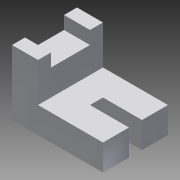
# Autodesk Inventor part: Aluminum
Saved by Autodesk Inventor 2015 (Build 190159000, 159)
## iProperties
Created: 2018-01-09
Part Number: Aluminum
Material: Aluminum 6061
Document SubType Name: Modeling
Designer: Administrator
Density: 2.7 g/cm^3
Appearance: Aluminum - Flat
Author: Administrator
Autodesk Inventor part; units mm, degrees
ref_plane "YZ Plane" through (0, 0, 0) normal (1, 0, 0) x (0, 1, 0)
ref_plane "XZ Plane" through (0, 0, 0) normal (0, 1, 0) x (-1, 0, 0)
ref_plane "XY Plane" through (0, 0, 0) normal (0, 0, 1) x (1, 0, 0)
sketch "Sketch1" plane through (0, 0, 0) normal (0, 0, 1) x (1, 0, 0)
  line L0 (0, 0) -> (0, 31.75)
  line L1 (0, 31.75) -> (12.7, 31.75)
  line L2 (12.7, 31.75) -> (12.7, 12.7)
  line L3 (12.7, 12.7) -> (44.45, 12.7)
  line L4 (44.45, 12.7) -> (44.45, 0)
  line L5 (44.45, 0) -> (0, 0)
  dimension "d0" = 31.75
  dimension "d1" = 44.45
  dimension "d2" = 19.05
  dimension "d3" = 12.7
  dimension "d4" = 12.7
  constraints: 12 end point, 4 perpendicular
  measures "d0" distance of L0.start L0.end
  measures "d1" distance of L4.end L0.start
  measures "d2" distance of L1.end L2.end
  measures "d3" distance of L0.end L1.end
  measures "d4" distance of L3.end L4.end
extrude "Extrusion1" add sketch "Sketch1" along normal blind 31.75
sketch "Sketch2" plane through (12.7, 12.7, 0) normal (1, 0, 0) x (0, 0, -1)
  line L0 (0, 19.05) -> (-31.75, 19.05) projected
  line L1 (-25.4, 19.05) -> (-25.4, 12.7)
  line L2 (-25.4, 12.7) -> (-6.35, 12.7)
  line L3 (-6.35, 12.7) -> (-6.35, 19.05)
  line L4 (-25.4, 19.05) -> (-6.35, 19.05)
  line L5 (-31.75, 0) -> (-31.75, 19.05) projected
  point P0 (0, -12.7)
  dimension "d7" = 6.35
  dimension "d8" = 19.05
  dimension "d9" = 6.35
  constraints: 8 end point, 4 perpendicular, 2 point on line
  measures "d7" distance of L2.end L3.end
  measures "d8" distance of L1.end L2.end
  measures "d9" distance between parallel lines of L1 L5
extrude "Extrusion2" cut sketch "Sketch2" against normal blind 31.75
sketch "Sketch3" plane through (44.45, 0, 0) normal (1, 0, 0) x (0, 0, -1)
  line L0 (-19.05, 12.7) -> (-19.05, 0)
  line L1 (-12.7, 0) -> (-12.7, 12.7)
  line L2 (-19.05, 12.7) -> (-12.7, 12.7)
  line L3 (-12.7, 0) -> (-19.05, 0)
  line L4 (-31.75, 0) -> (-31.75, 12.7) projected
  dimension "d12" = 12.7
  dimension "d13" = 12.7
  dimension "d16" = 6.35
  constraints: 8 end point, 1 perpendicular, 1 vertical
  measures "d12" distance between parallel lines of L4 L0
  measures "d13" distance of L1.start L1.end
  measures "d16" distance of L0.start L1.end
extrude "Extrusion3" cut sketch "Sketch3" against normal blind 19.05
body "Solid1"
